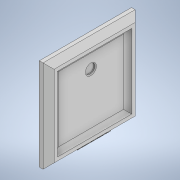
# Autodesk Inventor part: soporte
Saved by Autodesk Inventor 2021 (Build 250183000, 183)
## iProperties
Created: 2024-10-06
Part Number: soporte
Material: Generic
Document SubType Name: Modeling
Designer: hojan
Density: 1 g/cm^3
Appearance: Default
Author: hojan
Autodesk Inventor part; units mm, degrees
ref_plane "YZ Plane" through (0, 0, 0) normal (1, 0, 0) x (0, 1, 0)
ref_plane "XZ Plane" through (0, 0, 0) normal (0, 1, 0) x (-1, 0, 0)
ref_plane "XY Plane" through (0, 0, 0) normal (0, 0, 1) x (1, 0, 0)
sketch "Boceto1" plane through (0, 0, 0) normal (1, 0, 0) x (0, 1, 0)
  line L0 (-50, 50) -> (50, 50)
  line L1 (50, 50) -> (50, -50)
  line L2 (50, -50) -> (-50, -50)
  line L3 (-50, -50) -> (-50, 50)
  line L4 (-50, 50) -> (50, -50) construction
  line L5 (50, 50) -> (-50, -50) construction
  point P0 (0, 0)
  dimension "d0" = 100
  dimension "d1" = 100
  constraints: 12 end point, 2 midpoint, 2 parallel, 1 horizontal, 1 perpendicular
  measures "d0" distance of L1.end L2.end
  measures "d1" distance of L0.end L1.end
extrude "Extrusión1" add sketch "Boceto1" along normal blind 10
chamfer "Chaflán1" distance 6 angle 45 4 edges at (10, 50, 0) (10, 0, 50) (10, -50, 0) (10, 0, -50)
sketch "Boceto2" plane through (10, 0, 0) normal (1, 0, 0) x (0, 0, -1)
  line L0 (-40.25, -40.25) -> (40.25, -40.25)
  line L1 (40.25, -40.25) -> (40.25, 40.25)
  line L2 (40.25, 40.25) -> (-40.25, 40.25)
  line L3 (-40.25, 40.25) -> (-40.25, -40.25)
  line L4 (-40.25, -40.25) -> (40.25, 40.25) construction
  line L5 (40.25, -40.25) -> (-40.25, 40.25) construction
  point P0 (0, 0)
  dimension "d7" = 80.5
  dimension "d8" = 80.5
  constraints: 12 end point, 2 midpoint, 2 parallel, 1 horizontal, 1 perpendicular
  measures "d7" distance of L2.end L1.end
  measures "d8" distance of L1.end L0.end
extrude "Extrusión2" cut sketch "Boceto2" against normal blind 4
fillet "Empalme1" radius 5 4 edges at (6, 0, 40.25) (6, 40.25, 0) (6, -40.25, 0) (6, 0, -40.25)
sketch "Boceto3" plane through (6, 0, 0) normal (1, 0, 0) x (0, 0, -1)
  line L0 (0, 0) -> (0, 20)
  circle A0 centre (0, 20) radius 5
  dimension "d12" = 20
  dimension "d13" = 10
  constraints: 2 end point, 1 centre point, 1 coincident, 1 vertical
  measures "d12" distance of L0.start L0.end
  measures "d13" diameter of A0
extrude "Extrusión3" cut sketch "Boceto3" against normal blind 2
fillet "Empalme2" radius 1 1 edges at (6, 20, 5)
sketch "Boceto4" plane through (4, -50, 50) normal (0.7071068, -0.7071068, 0) x (-0.7071068, -0.7071068, 0)
  line L0 (-6.7253, 33.711) -> (-6.7253, 69.5066) construction
  line L1 (-6.7253, 69.5066) -> (-3.5588, 69.5066) construction
  line L2 (-3.5588, 69.5066) -> (-3.5588, 33.711) construction
  line L3 (-3.5588, 33.711) -> (-6.7253, 33.711) construction
  line L4 (-5.7084, 37.409) -> (-5.7084, 36.4228)
  line L5 (-5.7084, 36.4228) -> (-2.3031, 36.4228)
  spline S0 degree 2 poles (-2.3031, 36.4228) (-1.9757, 36.4228) (-1.6444, 36.1185) (-1.6444, 35.872) knots 0 0 0 1 2 2 2
  spline S1 degree 2 poles (-1.6444, 35.872) (-1.6444, 35.6254) (-1.9795, 35.3173) (-2.3031, 35.3173) knots 0 0 0 1 2 2 2
  line L6 (-2.3031, 35.3173) -> (-5.7084, 35.3173)
  line L7 (-5.7084, 35.3173) -> (-5.7084, 34.3311)
  spline S2 degree 2 poles (-5.7084, 34.3311) (-5.7084, 34.0538) (-5.9626, 33.7687) (-6.1783, 33.7687) knots 0 0 0 1 2 2 2
  spline S3 degree 2 poles (-6.1783, 33.7687) (-6.3902, 33.7687) (-6.6444, 34.0654) (-6.6444, 34.3311) knots 0 0 0 1 2 2 2
  line L8 (-6.6444, 34.3311) -> (-6.6444, 37.409)
  spline S4 degree 2 poles (-6.6444, 37.409) (-6.6444, 37.6902) (-6.3825, 37.9752) (-6.1783, 37.9752) knots 0 0 0 1 2 2 2
  spline S5 degree 2 poles (-6.1783, 37.9752) (-5.9665, 37.9752) (-5.7084, 37.6863) (-5.7084, 37.409) knots 0 0 0 1 2 2 2
  line L9 (-6.0743, 39.6123) -> (-4.7685, 39.6123)
  line L10 (-4.7685, 39.6123) -> (-4.7685, 41.5654)
  line L11 (-4.7685, 41.5654) -> (-6.0743, 41.5654)
  spline S6 degree 2 poles (-6.0743, 41.5654) (-6.3902, 41.5654) (-6.7253, 41.8658) (-6.7253, 42.1123) knots 0 0 0 1 2 2 2
  spline S7 degree 2 poles (-6.7253, 42.1123) (-6.7253, 42.3627) (-6.394, 42.6709) (-6.0743, 42.6709) knots 0 0 0 1 2 2 2
  line L12 (-6.0743, 42.6709) -> (-2.3031, 42.6709)
  spline S8 degree 2 poles (-2.3031, 42.6709) (-1.9795, 42.6709) (-1.6444, 42.3589) (-1.6444, 42.1123) knots 0 0 0 1 2 2 2
  spline S9 degree 2 poles (-1.6444, 42.1123) (-1.6444, 41.862) (-1.9834, 41.5654) (-2.3031, 41.5654) knots 0 0 0 1 2 2 2
  line L13 (-2.3031, 41.5654) -> (-3.844, 41.5654)
  line L14 (-3.844, 41.5654) -> (-3.844, 39.6123)
  line L15 (-3.844, 39.6123) -> (-2.3031, 39.6123)
  spline S10 degree 2 poles (-2.3031, 39.6123) (-1.9795, 39.6123) (-1.6444, 39.3003) (-1.6444, 39.0538) knots 0 0 0 1 2 2 2
  spline S11 degree 2 poles (-1.6444, 39.0538) (-1.6444, 38.8034) (-1.9834, 38.5068) (-2.3031, 38.5068) knots 0 0 0 1 2 2 2
  line L16 (-2.3031, 38.5068) -> (-6.0743, 38.5068)
  spline S12 degree 2 poles (-6.0743, 38.5068) (-6.3902, 38.5068) (-6.7253, 38.7996) (-6.7253, 39.0538) knots 0 0 0 1 2 2 2
  spline S13 degree 2 poles (-6.7253, 39.0538) (-6.7253, 39.3042) (-6.394, 39.6123) (-6.0743, 39.6123) knots 0 0 0 1 2 2 2
  line L17 (-5.7623, 46.9043) -> (-5.7623, 44.7895)
  line L18 (-5.7623, 44.7895) -> (-4.7222, 44.7895)
  line L19 (-4.7222, 44.7895) -> (-4.7222, 46.731)
  spline S14 degree 2 poles (-4.7222, 46.731) (-4.7222, 46.9814) (-4.4834, 47.2395) (-4.2946, 47.2395) knots 0 0 0 1 2 2 2
  spline S15 degree 2 poles (-4.2946, 47.2395) (-4.102, 47.2395) (-3.8555, 46.9852) (-3.8555, 46.731) knots 0 0 0 1 2 2 2
  line L20 (-3.8555, 46.731) -> (-3.8555, 44.7895)
  line L21 (-3.8555, 44.7895) -> (-2.6306, 44.7895)
  line L22 (-2.6306, 44.7895) -> (-2.6306, 46.9775)
  spline S16 degree 2 poles (-2.6306, 46.9775) (-2.6306, 47.2356) (-2.3802, 47.5091) (-2.176, 47.5091) knots 0 0 0 1 2 2 2
  spline S17 degree 2 poles (-2.176, 47.5091) (-1.9757, 47.5091) (-1.7253, 47.2356) (-1.7253, 46.9775) knots 0 0 0 1 2 2 2
  line L23 (-1.7253, 46.9775) -> (-1.7253, 44.3466)
  spline S18 degree 2 poles (-1.7253, 44.3466) (-1.7253, 43.9999) (-2.045, 43.684) (-2.3879, 43.684) knots 0 0 0 1 2 2 2
  line L24 (-2.3879, 43.684) -> (-5.9857, 43.684)
  spline S19 degree 2 poles (-5.9857, 43.684) (-6.2091, 43.684) (-6.5057, 43.8227) (-6.6444, 44.1231) (-6.6444, 44.3466) knots 0 0 0 1 2 3 3 3
  line L25 (-6.6444, 44.3466) -> (-6.6444, 46.9043)
  spline S20 degree 2 poles (-6.6444, 46.9043) (-6.6444, 47.1624) (-6.4017, 47.4282) (-6.2053, 47.4282) knots 0 0 0 1 2 2 2
  spline S21 degree 2 poles (-6.2053, 47.4282) (-6.005, 47.4282) (-5.7623, 47.1624) (-5.7623, 46.9043) knots 0 0 0 1 2 2 2
  spline S22 degree 2 poles (-3.3047, 54.1501) (-3.0658, 54.1501) (-2.5073, 53.9151) (-1.9757, 53.4144) (-1.6444, 52.6362) (-1.6444, 52.1239) knots 0 0 0 1 2 3 4 4 4
  spline S23 degree 2 poles (-1.6444, 52.1239) (-1.6444, 51.7348) (-1.7908, 51.0993) (-2.1067, 50.5715) (-2.3648, 50.3558) knots 0 0 0 1 2 3 3 3
  spline S24 degree 2 poles (-2.3648, 50.3558) (-2.5959, 50.1593) (-3.1698, 49.882) (-3.8131, 49.7472) (-4.1791, 49.7472) knots 0 0 0 1 2 3 3 3
  spline S25 degree 2 poles (-4.1791, 49.7472) (-4.7723, 49.7472) (-5.7045, 50.09) (-6.3748, 50.7372) (-6.7253, 51.6077) (-6.7253, 52.0969) knots 0 0 0 1 2 3 4 4 4
  spline S26 degree 2 poles (-6.7253, 52.0969) (-6.7253, 52.694) (-6.2438, 53.6339) (-5.5312, 54.1385) (-5.2114, 54.1385) knots 0 0 0 1 2 3 3 3
  spline S27 degree 2 poles (-5.2114, 54.1385) (-5.0188, 54.1385) (-4.7222, 53.865) (-4.7222, 53.6686) knots 0 0 0 1 2 2 2
  spline S28 degree 2 poles (-4.7222, 53.6686) (-4.7222, 53.4529) (-4.9225, 53.241) (-5.1498, 53.1177) knots 0 0 0 1 2 2 2
  spline S29 degree 2 poles (-5.1498, 53.1177) (-5.4888, 52.9367) (-5.8201, 52.4552) (-5.8201, 52.1046) knots 0 0 0 1 2 2 2
  spline S30 degree 2 poles (-5.8201, 52.1046) (-5.8201, 51.5422) (-4.9572, 50.8681) (-4.1483, 50.8681) knots 0 0 0 1 2 2 2
  spline S31 degree 2 poles (-4.1483, 50.8681) (-3.5974, 50.8681) (-2.8925, 51.1686) (-2.5497, 51.7079) (-2.5497, 52.07) knots 0 0 0 1 2 3 3 3
  spline S32 degree 2 poles (-2.5497, 52.07) (-2.5497, 52.4667) (-2.9387, 53.006) (-3.3509, 53.1563) knots 0 0 0 1 2 2 2
  spline S33 degree 2 poles (-3.3509, 53.1563) (-3.5165, 53.214) (-3.7939, 53.4221) (-3.7939, 53.6609) knots 0 0 0 1 2 2 2
  spline S34 degree 2 poles (-3.7939, 53.6609) (-3.7939, 53.8612) (-3.5088, 54.1501) (-3.3047, 54.1501) knots 0 0 0 1 2 2 2
  line L26 (-3.7708, 54.9976) -> (-6.0743, 54.9976)
  spline S35 degree 2 poles (-6.0743, 54.9976) (-6.3902, 54.9976) (-6.7253, 55.298) (-6.7253, 55.5446) knots 0 0 0 1 2 2 2
  spline S36 degree 2 poles (-6.7253, 55.5446) (-6.7253, 55.8026) (-6.3902, 56.1031) (-6.0743, 56.1031) knots 0 0 0 1 2 2 2
  line L27 (-6.0743, 56.1031) -> (-3.7207, 56.1031)
  spline S37 degree 2 poles (-3.7207, 56.1031) (-3.3278, 56.1031) (-2.8232, 56.2726) (-2.5497, 56.6886) (-2.5497, 57.0815) knots 0 0 0 1 2 3 3 3
  spline S38 degree 2 poles (-2.5497, 57.0815) (-2.5497, 57.6131) (-3.1082, 58.0484) (-3.7014, 58.0484) knots 0 0 0 1 2 2 2
  line L28 (-3.7014, 58.0484) -> (-6.0743, 58.0484)
  spline S39 degree 2 poles (-6.0743, 58.0484) (-6.394, 58.0484) (-6.7253, 58.345) (-6.7253, 58.5954) knots 0 0 0 1 2 2 2
  spline S40 degree 2 poles (-6.7253, 58.5954) (-6.7253, 58.8458) (-6.394, 59.154) (-6.0743, 59.154) knots 0 0 0 1 2 2 2
  line L29 (-6.0743, 59.154) -> (-3.7708, 59.154)
  spline S41 degree 2 poles (-3.7708, 59.154) (-3.2045, 59.154) (-2.4225, 58.9267) (-2.1259, 58.6108) knots 0 0 0 1 2 2 2
  spline S42 degree 2 poles (-2.1259, 58.6108) (-1.8755, 58.3373) (-1.6444, 57.6208) (-1.6444, 57.1509) knots 0 0 0 1 2 2 2
  spline S43 degree 2 poles (-1.6444, 57.1509) (-1.6444, 56.5846) (-1.891, 55.7641) (-2.4148, 55.2402) (-3.2161, 54.9976) (-3.7708, 54.9976) knots 0 0 0 1 2 3 4 4 4
  line L30 (-1.7253, 62.2857) -> (-1.7253, 60.8258)
  spline S44 degree 2 poles (-1.7253, 60.8258) (-1.7253, 60.4752) (-2.0489, 60.167) (-2.3879, 60.167) knots 0 0 0 1 2 2 2
  line L31 (-2.3879, 60.167) -> (-5.9857, 60.167)
  spline S45 degree 2 poles (-5.9857, 60.167) (-6.3285, 60.167) (-6.6444, 60.4829) (-6.6444, 60.8258) knots 0 0 0 1 2 2 2
  line L32 (-6.6444, 60.8258) -> (-6.6444, 62.3743)
  spline S46 degree 2 poles (-6.6444, 62.3743) (-6.6444, 62.721) (-6.5558, 63.2449) (-6.3902, 63.4875) knots 0 0 0 1 2 2 2
  spline S47 degree 2 poles (-6.3902, 63.4875) (-6.3208, 63.6339) (-5.9934, 63.9113) (-5.5967, 64.0576) (-5.3771, 64.0576) knots 0 0 0 1 2 3 3 3
  spline S48 degree 2 poles (-5.3771, 64.0576) (-4.6144, 64.0576) (-4.337, 63.3373) knots 0 0 0 1 1 1
  spline S49 degree 2 poles (-4.337, 63.3373) (-4.0751, 64.2811) (-3.1583, 64.2811) knots 0 0 0 1 1 1
  spline S50 degree 2 poles (-3.1583, 64.2811) (-2.7384, 64.2811) (-2.0604, 63.8458) (-1.891, 63.449) knots 0 0 0 1 2 2 2
  spline S51 degree 2 poles (-1.891, 63.449) (-1.8024, 63.2526) (-1.7253, 62.6748) (-1.7253, 62.2857) knots 0 0 0 1 2 2 2
  line L33 (-3.8517, 62.2125) -> (-3.8517, 61.2726)
  line L34 (-3.8517, 61.2726) -> (-2.5882, 61.2726)
  line L35 (-2.5882, 61.2726) -> (-2.5882, 62.2472)
  spline S52 degree 2 poles (-2.5882, 62.2472) (-2.5882, 63.1601) (-3.2315, 63.1601) knots 0 0 0 1 1 1
  spline S53 degree 2 poles (-3.2315, 63.1601) (-3.555, 63.1601) (-3.8517, 62.6979) (-3.8517, 62.2125) knots 0 0 0 1 2 2 2
  line L36 (-5.7816, 61.2726) -> (-4.6799, 61.2726)
  line L37 (-4.6799, 61.2726) -> (-4.6799, 62.0931)
  spline S54 degree 2 poles (-4.6799, 62.0931) (-4.6799, 62.4436) (-4.8031, 62.8019) (-4.9572, 62.8866) knots 0 0 0 1 2 2 2
  spline S55 degree 2 poles (-4.9572, 62.8866) (-5.0959, 62.9675) (-5.25, 62.9675) knots 0 0 0 1 1 1
  spline S56 degree 2 poles (-5.25, 62.9675) (-5.5658, 62.9675) (-5.7816, 62.5014) (-5.7816, 61.9891) knots 0 0 0 1 2 2 2
  line L38 (-5.7816, 61.9891) -> (-5.7816, 61.2726)
  line L39 (-5.7623, 68.3026) -> (-5.7623, 66.1878)
  line L40 (-5.7623, 66.1878) -> (-4.7222, 66.1878)
  line L41 (-4.7222, 66.1878) -> (-4.7222, 68.1293)
  spline S57 degree 2 poles (-4.7222, 68.1293) (-4.7222, 68.3797) (-4.4834, 68.6378) (-4.2946, 68.6378) knots 0 0 0 1 2 2 2
  spline S58 degree 2 poles (-4.2946, 68.6378) (-4.102, 68.6378) (-3.8555, 68.3835) (-3.8555, 68.1293) knots 0 0 0 1 2 2 2
  line L42 (-3.8555, 68.1293) -> (-3.8555, 66.1878)
  line L43 (-3.8555, 66.1878) -> (-2.6306, 66.1878)
  line L44 (-2.6306, 66.1878) -> (-2.6306, 68.3758)
  spline S59 degree 2 poles (-2.6306, 68.3758) (-2.6306, 68.6339) (-2.3802, 68.9074) (-2.176, 68.9074) knots 0 0 0 1 2 2 2
  spline S60 degree 2 poles (-2.176, 68.9074) (-1.9757, 68.9074) (-1.7253, 68.6339) (-1.7253, 68.3758) knots 0 0 0 1 2 2 2
  line L45 (-1.7253, 68.3758) -> (-1.7253, 65.7449)
  spline S61 degree 2 poles (-1.7253, 65.7449) (-1.7253, 65.3982) (-2.045, 65.0823) (-2.3879, 65.0823) knots 0 0 0 1 2 2 2
  line L46 (-2.3879, 65.0823) -> (-5.9857, 65.0823)
  spline S62 degree 2 poles (-5.9857, 65.0823) (-6.2091, 65.0823) (-6.5057, 65.221) (-6.6444, 65.5214) (-6.6444, 65.7449) knots 0 0 0 1 2 3 3 3
  line L47 (-6.6444, 65.7449) -> (-6.6444, 68.3026)
  spline S63 degree 2 poles (-6.6444, 68.3026) (-6.6444, 68.5607) (-6.4017, 68.8265) (-6.2053, 68.8265) knots 0 0 0 1 2 2 2
  spline S64 degree 2 poles (-6.2053, 68.8265) (-6.005, 68.8265) (-5.7623, 68.5607) (-5.7623, 68.3026) knots 0 0 0 1 2 2 2
  point P0 (-32.5269, 50)
  constraints: 2 other
extrude "Extrusión4" add sketch "Boceto4" along normal blind 0.5
